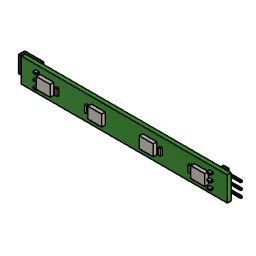
ERCF Carrot on a Stick v2 (Autodesk Fusion 360 design; units mm, degrees)
Autodesk Fusion 360 part; units mm, degrees
note: some values were not read from the file. Chosen so that the rebuilt part matches the saved one: which bodies a step acts on.
sketch "Back" plane through (0, 0, 0) normal (0, 1, 0) x (1, 0, 0)
  line L0 (46.15, 5.45) -> (-46.15, 5.45)
  line L1 (-46.15, 5.45) -> (-46.15, -5.45)
  line L2 (-46.15, -5.45) -> (46.15, -5.45)
  line L3 (46.15, -5.45) -> (46.15, 5.45)
  line L4 (46.15, 5.45) -> (-46.15, -5.45) construction
  line L5 (-46.15, 5.45) -> (46.15, -5.45) construction
  line L6 (38.1, -3.375) -> (49.5, -3.375)
  line L7 (49.5, -3.375) -> (49.5, 3.375)
  line L8 (49.5, 3.375) -> (38.1, 3.375)
  line L9 (38.1, 3.375) -> (38.1, -3.375)
  line L10 (46.15, 0) -> (49.5, 0) construction
  line L11 (-49.05, -3.75) -> (-37.95, -3.75)
  line L12 (-37.95, -3.75) -> (-37.95, 3.75)
  line L13 (-37.95, 3.75) -> (-49.05, 3.75)
  line L14 (-49.05, 3.75) -> (-49.05, -3.75)
  line L15 (-46.15, 0) -> (-49.05, 0) construction
  line L16 (49.5, 0) -> (38.1, 0) construction
  line L17 (38.1, -2.725) -> (49.5, -2.725)
  line L18 (49.5, 2.725) -> (38.1, 2.725)
  line L19 (49.5, -0.325) -> (38.1, -0.325)
  line L20 (49.5, 0.325) -> (38.1, 0.325)
  line L21 (42.65, -3.375) -> (42.65, 3.375)
  line L22 (40.15, -3.375) -> (40.15, 3.375)
  line L23 (39.75, 3.375) -> (39.75, -3.375)
  line L24 (42.65, -3.75) -> (40.1, -3.75)
  line L25 (40.1, -3.75) -> (40.1, 3.75)
  line L26 (40.1, 3.75) -> (42.65, 3.75)
  line L27 (42.65, 3.75) -> (42.65, -3.75)
  line L28 (-40.5, 3.75) -> (-40.5, -3.75)
  dimension "d1" = 92.3
  dimension "d2" = 10.9
  dimension "d3" = 11.4
  dimension "d4" = 6.75
  dimension "d5" = 3.35
  dimension "d6" = 11.1
  dimension "d7" = 7.5
  dimension "d8" = 2.9
  dimension "d25" = -0.65
  dimension "d26" = -0.65
  dimension "d27" = -0.325
  dimension "d28" = 0.325
  dimension "d29" = -6.85
  dimension "d30" = -9.35
  dimension "d36" = -1.65
  dimension "d42" = 2.55
  dimension "d43" = 7.5
  dimension "d46" = -8.55
  constraint horizontal L0
  constraint perpendicular L0 L1
  constraint parallel L0 L2
  constraint parallel L1 L3
  constraint coincident L4 origin
  constraint coincident L5 origin
  constraint horizontal L6
  constraint vertical L7
  constraint horizontal L8
  constraint vertical L9
  constraint midpoint L3 L10.start
  constraint perpendicular L9 L10
  constraint midpoint L7 L10.end
  constraint horizontal L11
  constraint vertical L12
  constraint horizontal L13
  constraint vertical L14
  constraint midpoint L1 L15.start
  constraint perpendicular L1 L15
  constraint midpoint L14 L15.end
  constraint midpoint L9 L16.end
  constraint horizontal L24
  constraint vertical L25
  constraint horizontal L26
  constraint vertical L27
  constraint midpoint L21 L27
  measures "d1" distance of L1.end L2.end
  measures "d2" distance of L0.end L1.end
  measures "d3" distance of L6.start L6.end
  measures "d4" distance of L6.start L8.end
  measures "d5" distance of L10.start L10.end
  measures "d6" distance of L11.start L11.end
  measures "d7" distance of L11.start L13.end
  measures "d8" distance of L15.start L15.end
  measures "d42" distance of L24.start L24.end
  measures "d43" distance of L24.start L26.end
sketch "LEDs" plane through (0, 0, 0) normal (0, 1, 0) x (1, 0, 0)
  line L0 (-46.15, -5.45) -> (46.15, -5.45)
  line L1 (46.15, 5.45) -> (-46.15, 5.45)
  line L2 (-46.15, 5.45) -> (-46.15, -5.45)
  line L3 (46.15, -5.45) -> (46.15, 5.45)
  line L4 (-37.8, -2.5) -> (-31.55, -2.5)
  line L5 (-31.55, -2.5) -> (-31.55, 2.5)
  line L6 (-31.55, 2.5) -> (-37.8, 2.5)
  line L7 (-37.8, 2.5) -> (-37.8, -2.5)
  line L8 (-46.15, 0) -> (-37.8, 0) construction
  line L9 (-8.5, -2.5) -> (-8.5, 2.5)
  line L10 (-14.75, 2.5) -> (-14.75, -2.5)
  line L11 (-14.75, -2.5) -> (-8.5, -2.5)
  line L12 (-8.5, 2.5) -> (-14.75, 2.5)
  line L13 (14.55, -2.5) -> (14.55, 2.5)
  line L14 (8.3, 2.5) -> (8.3, -2.5)
  line L15 (8.3, -2.5) -> (14.55, -2.5)
  line L16 (14.55, 2.5) -> (8.3, 2.5)
  line L17 (37.6, -2.5) -> (37.6, 2.5)
  line L18 (31.35, 2.5) -> (31.35, -2.5)
  line L19 (31.35, -2.5) -> (37.6, -2.5)
  line L20 (37.6, 2.5) -> (31.35, 2.5)
  dimension "d9" = 6.25
  dimension "d10" = 5
  dimension "d11" = 8.35
  dimension "d14" = 23.05
  dimension "d15" = 0
  constraint horizontal L4
  constraint vertical L5
  constraint horizontal L6
  constraint vertical L7
  constraint midpoint L2 L8.start
  constraint perpendicular L2 L8
  constraint midpoint L7 L8.end
  measures "d9" distance of L4.start L4.end
  measures "d10" distance of L4.start L6.end
  measures "d11" distance of L8.start L8.end
sketch "Capacitors" plane through (0, 0, 0) normal (0, 1, 0) x (1, 0, 0)
  line L0 (-30.3, -1.5) -> (-29.3, -1.5)
  line L1 (-29.3, -1.5) -> (-29.3, 1.5)
  line L2 (-29.3, 1.5) -> (-30.3, 1.5)
  line L3 (-30.3, 1.5) -> (-30.3, -1.5)
  line L4 (-37.8, 2.5) -> (-37.8, -2.5) construction
  line L5 (-8.5, -2.5) -> (-8.5, 2.5) construction
  line L6 (-37.8, 0) -> (-30.3, 0) construction
  line L7 (-8.5, 0) -> (-16, 0) construction
  line L8 (-17, -1.5) -> (-16, -1.5)
  line L9 (-16, -1.5) -> (-16, 1.5)
  line L10 (-16, 1.5) -> (-17, 1.5)
  line L11 (-17, 1.5) -> (-17, -1.5)
  line L12 (0, -1.75) -> (0, -22.5)
  line L13 (29.3, -1.5) -> (29.3, 1.5)
  line L14 (29.3, 1.5) -> (30.3, 1.5)
  line L15 (30.3, 1.5) -> (30.3, -1.5)
  line L16 (30.3, -1.5) -> (29.3, -1.5)
  line L17 (17, 1.5) -> (17, -1.5)
  line L18 (16, -1.5) -> (16, 1.5)
  line L19 (17, -1.5) -> (16, -1.5)
  line L20 (16, 1.5) -> (17, 1.5)
  line L21 (-46.15, -5.45) -> (46.15, -5.45)
  line L22 (46.15, 5.45) -> (-46.15, 5.45)
  line L23 (-46.15, 5.45) -> (-46.15, -5.45)
  line L24 (46.15, -5.45) -> (46.15, 5.45)
  dimension "d19" = 1
  dimension "d20" = 3
  dimension "d21" = 7.5
  dimension "d22" = 7.5
  dimension "d23" = 1
  dimension "d24" = 3
  constraint horizontal L0
  constraint vertical L1
  constraint horizontal L2
  constraint vertical L3
  constraint midpoint L4 L6.start
  constraint perpendicular L4 L6
  constraint midpoint L5 L7.start
  constraint perpendicular L5 L7
  constraint midpoint L3 L6.end
  constraint horizontal L8
  constraint vertical L9
  constraint horizontal L10
  constraint vertical L11
  constraint midpoint L7.end L9
  constraint symmetric L0.start L12 L15.end
  constraint symmetric L0.end L12 L13.start
  constraint symmetric L1.end L12 L13.end
  constraint symmetric L2.end L12 L14.end
  constraint symmetric L8.start L12 L17.end
  constraint symmetric L8.end L12 L18.start
  constraint symmetric L9.end L12 L18.end
  constraint symmetric L10.end L12 L17.start
  measures "d19" distance of L0.start L0.end
  measures "d20" distance of L0.start L2.end
  measures "d21" distance of L6.start L6.end
  measures "d22" distance of L7.start L7.end
  measures "d23" distance of L8.start L8.end
  measures "d24" distance of L8.start L10.end
extrude "Extrude1" add sketch "Back" against normal blind 1.7 contours L0 L1 L2 L3 L6 L8 L9 L11 L12 L13 L24 L25 L26 L27 | L3 L8 L18 L21 L27 | L1 L11 L13 L28 | L3 L18 L20 L21 L27 | L8 L18 L21 L22 L27 | L8 L25 L26 L27 | L11 L12 L13 L28 | L3 L19 L20 L21 L27 | L18 L20 L21 L22 L27 | L8 L18 L22 L25 | L3 L17 L19 L21 L27 | L19 L20 L21 L22 L27 | L18 L20 L22 L25 | L8 L18 L23 L25 | L3 L6 L17 L21 L27 | L17 L19 L21 L22 L27 | L19 L20 L22 L25 | L18 L20 L23 L25 | L8 L9 L18 L23 | L6 L17 L21 L22 L27 | L17 L19 L22 L25 | L19 L20 L23 L25 | L9 L18 L20 L23 | L6 L24 L25 L27 | L6 L17 L22 L25 | L17 L19 L23 L25 | L9 L19 L20 L23 | L6 L17 L23 L25 | L9 L17 L19 L23 | L6 L9 L17 L23 makes body 1
extrude "Extrude2" add sketch "Back" along normal blind 0.65 from surface at 1 separate body contours L3 L7 L8 L18 | L3 L8 L18 L21 L27 | L8 L18 L21 L22 L27 | L3 L7 L19 L20 | L3 L19 L20 L21 L27 | L8 L18 L22 L25 | L19 L20 L21 L22 L27 | L8 L18 L23 L25 | L3 L6 L7 L17 | L3 L6 L17 L21 L27 | L19 L20 L22 L25 | L8 L9 L18 L23 | L6 L17 L21 L22 L27 | L19 L20 L23 L25 | L6 L17 L22 L25 | L9 L19 L20 L23 | L6 L17 L23 L25 | L6 L9 L17 L23 makes body 2 at (45.7, 1, 3.1583) makes body 3 at (45.7, 1, 0.1083) makes body 4 at (41.9, 1.2167, -2.725)
extrude "Extrude3" add sketch "Back" against normal blind 4.5 from surface at 1.65 contours L8 L9 L18 L23 | L9 L19 L20 L23 | L6 L9 L17 L23 bodies 3 4 2
mirror "Mirror1" about plane through (0, 0, 0) normal (1, 0, 0) of bodies 4 3 2 makes body 5 at (-38.65, -0.0667, 3.375) makes body 6 at (-38.65, -0.0667, -0.325) makes body 7 at (-38.65, -0.0667, -2.725)
combine "Combine2" operation cut target body 1 tool bodies 2 3 4 7 6 5 keep tools
split "Split1" by curves path "Back" along L28 bodies 5 6 7 makes body 10 at (-43.5, 1.65, -3.1583) makes body 9 at (-46.5, 1.65, 0.1083) makes body 8 at (-46.5, 1.65, 3.1583)
delete_body "RemoveBody1" bodies 8
delete_body "RemoveBody2" bodies 9
delete_body "RemoveBody3" bodies 10
extrude "Extrude5" add sketch "Back" along normal blind 2.75 separate body contours L1 L11 L13 L28 | L1 L11 L13 L14 makes body 11
copy_body "Body->Comp1" bodies 1 removing the originals makes body 12 in component "LED PCB"
copy_body "CutPasteBodies1" bodies 11 2 5 6 4 3 7 removing the originals makes body 13 makes body 14 makes body 15 makes body 16 makes body 17 makes body 18 makes body 19 in component "LED PCB"
extrude "Extrude1'" add sketch "LEDs" against normal blind 1.6 from surface at -1.7 separate body contours L4 L5 L6 L7 | L9 L10 L11 L12 | L13 L14 L15 L16 | L17 L18 L19 L20 makes body 20 at (-10.5833, -1.7, 0.8333) makes body 21 at (12.4667, -1.7, 0.8333) makes body 22 at (-35.7167, -1.7, -0.8333) makes body 23 at (35.5167, -1.7, 0.8333) in component "LEDs"
extrude "Extrude1''" add sketch "Capacitors" against normal blind 0.8 from surface at -1.7 separate body contours L0 L1 L2 L3 | L8 L9 L10 L11 | L13 L14 L15 L16 | L17 L18 L19 L20 makes body 24 at (29.9667, -1.7, 0.5) makes body 25 at (-16.6667, -1.7, -0.5) makes body 26 at (-29.9667, -1.7, 0.5) makes body 27 at (16.3333, -1.7, -0.5) in component "Capacitors"
sketch "Header Comb" plane through (0, 0, 0) normal (1, 0, 0) x (0, 1, 0)
  line L0 (1, 3.375) -> (1, 2.725)
  line L1 (1, 2.725) -> (1.65, 2.725)
  line L2 (1.65, 2.725) -> (1.65, 3.375)
  line L3 (1.65, 3.375) -> (1, 3.375)
  line L4 (1, 0.325) -> (1, -0.325)
  line L5 (1, -0.325) -> (1.65, -0.325)
  line L6 (1.65, -0.325) -> (1.65, 0.325)
  line L7 (1.65, 0.325) -> (1, 0.325)
  line L8 (1, -2.725) -> (1, -3.375)
  line L9 (1, -3.375) -> (1.65, -3.375)
  line L10 (1.65, -3.375) -> (1.65, -2.725)
  line L11 (1.65, -2.725) -> (1, -2.725)
  line L12 (0.075, 4.1) -> (2.575, 4.1)
  line L13 (2.575, 4.1) -> (2.575, -4.1)
  line L14 (2.575, -4.1) -> (0.075, -4.1)
  line L15 (0.075, -4.1) -> (0.075, 4.1)
  line L16 (1.325, 4.1) -> (1.325, -4.1) construction
  line L17 (1, 0.325) -> (1.65, -0.325) construction
  dimension "d55" = 2.5
  dimension "d56" = 8.2
  constraint horizontal L12
  constraint vertical L13
  constraint horizontal L14
  constraint vertical L15
  constraint midpoint L12 L16.start
  constraint midpoint L14 L16.end
  constraint coincident L4.start L7.end
  constraint coincident L5.end L6.start
  constraint midpoint L16 L17
  measures "d55" distance of L12.start L12.end
  measures "d56" distance of L12.start L14.end
extrude "Extrude6" add sketch "Header Comb" along normal blind 2.5 from surface at 40.15 separate body makes body 28
copy_body "CutPasteBodies2" bodies 28 removing the originals makes body 29 in component "LED PCB"
copy_body "Body->Comp1'" bodies 12 removing the originals makes body 30 in component "PCB"
copy_body "Body->Comp2" bodies 13 removing the originals makes body 31 in component "Connector"
copy_body "Body->Comp3" bodies 29 removing the originals makes body 32 in component "Header Comb"
copy_body "Body->Comp4" bodies 15 removing the originals makes body 33 in component "Header 1"
copy_body "CutPasteBodies1'" bodies 19 removing the originals makes body 34 in component "Header 1"
copy_body "CutPasteBodies2'" bodies 16 removing the originals makes body 35 in component "Header 1"
copy_body "Body->Comp5" bodies 14 removing the originals makes body 36 in component "Header 2"
copy_body "CutPasteBodies1''" bodies 17 18 removing the originals makes body 37 makes body 38 in component "Header 2"
component "LED PCB" placed x (1, 0, 0) y (0, 1, 0) z (0, 0, 1) at (0, 0, 0)
component "LEDs" placed x (1, 0, 0) y (0, 1, 0) z (0, 0, 1) at (0, 0, 0) in component "LED PCB"
component "Capacitors" placed x (1, 0, 0) y (0, 1, 0) z (0, 0, 1) at (0, 0, 0) in component "LED PCB"
component "PCB" placed x (1, 0, 0) y (0, 1, 0) z (0, 0, 1) at (0, 0, 0) in component "LED PCB"
component "Connector" placed x (1, 0, 0) y (0, 1, 0) z (0, 0, 1) at (0, 0, 0) in component "LED PCB"
component "Header Comb" placed x (1, 0, 0) y (0, 1, 0) z (0, 0, 1) at (0, 0, 0) in component "LED PCB"
component "Header 1" placed x (1, 0, 0) y (0, 1, 0) z (0, 0, 1) at (0, 0, 0) in component "LED PCB"
component "Header 2" placed x (1, 0, 0) y (0, 1, 0) z (0, 0, 1) at (0, 0, 0) in component "LED PCB"
equation "d26 = d25"
equation "d27 = d25 / 2"
equation "d28 = -d25 / 2"
equation "d29 = -d5 - 3.5 mm"
equation "d30 = d29 - 2.5 mm"
equation "d50 = 0.00 mm - 1.6 mm"
